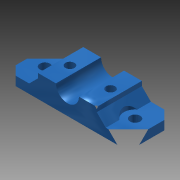
# Autodesk Inventor part: ZAxisRodClampBody
Saved by Autodesk Inventor 2015 SP1 (Build 190203100, 203)
## iProperties
Created: 2014-08-22
Part Number: ZAxisRodClampBody
Material: ABS Plastic
Document SubType Name: Modeling
Designer: t_clevj
Density: 1.06 g/cm^3
Appearance: Cyan
Mass: 6.86404 g
Surface Area: 36.706 cm^2
Volume: 6.47551 cm^3
Author: t_clevj
Autodesk Inventor part; units mm, degrees
ref_plane "YZ Plane" through (0, 0, 0) normal (1, 0, 0) x (0, 1, 0)
ref_plane "XZ Plane" through (0, 0, 0) normal (0, 1, 0) x (-1, 0, 0)
ref_plane "XY Plane" through (0, 0, 0) normal (0, 0, 1) x (1, 0, 0)
sketch "Sketch1" plane through (0, 0, 0) normal (0, 0, 1) x (1, 0, 0)
  circle A0 centre (0, 0) radius 2.25
  circle A1 centre (40, 0) radius 2.25
  line L0 (-7, 10) -> (47, 10)
  line L1 (-7, -10) -> (47, -10)
  line L2 (-7, -10) -> (-7, 10)
  line L3 (47, 10) -> (47, -10)
  dimension "d0" = 4.5
  dimension "d1" = 4.5
  dimension "d2" = 40
  dimension "d48" = 7
  dimension "d49" = 7
  dimension "d50" = 20
  dimension "d51" = 10
  constraints: 8 end point, 2 centre point, 2 perpendicular, 2 vertical, 1 coincident, 1 horizontal alignment
  measures "d0" diameter of A0
  measures "d1" diameter of A1
  measures "d2" distance of A1.centre point (0, 0)
  measures "d48" distance from line of A1.centre L3
  measures "d49" distance from line of L2 point (0, 0)
  measures "d50" distance between parallel lines of L1 L0
  measures "d51" distance from line of L0 A1.centre
extrude "Extrusion1" add sketch "Sketch1" along normal blind 4
ref_plane "Work Plane1" through (-7, 0, 0) normal (0, 1, 0) x (1, 0, 0)
sketch "Sketch4" plane through (-7, 0, 0) normal (0, 1, 0) x (1, 0, 0)
  line L0 (0, 0) -> (54, 0) projected
  line L1 (0, 0) -> (0, -4) projected
  line L2 (54, -4) -> (0, -4) projected
  line L3 (54, 0) -> (54, -4) projected
  line L4 (0, 0) -> (0, 0) projected
  line L5 (0, 0) -> (0, -4) projected
  line L6 (0, -4) -> (0, -4) projected
  line L7 (0, 0) -> (0, -4) projected
  line L8 (40, 0) -> (40, 0) projected
  line L9 (40, 0) -> (40, -4) projected
  line L10 (40, -4) -> (40, -4) projected
  line L11 (40, 0) -> (40, -4) projected
  circle A0 centre (27, -10) radius 5.1
  line L12 (14, -4) -> (14, -10)
  line L13 (14, -10) -> (21.9, -10)
  line L14 (32.1, -10) -> (40, -10)
  line L15 (40, -10) -> (40, -4)
  line L16 (0, -4) -> (54, -4) projected
  line L17 (14, -4) -> (40, -4)
  point P0 (7, 0)
  dimension "d23" = 10.2
  dimension "d24" = 6
  dimension "d25" = 26
  dimension "d26" = 13
  dimension "d27" = 14
  constraints: 10 end point, 4 point on line, 2 perpendicular, 2 point on circle, 1 centre point, 1 collinear, 1 horizontal alignment, 1 vertical
  measures "d23" diameter of A0
  measures "d24" distance from line of L2 A0.centre
  measures "d25" distance between parallel lines of L12 L15
  measures "d26" distance from line of A0.centre L15
  measures "d27" distance between parallel lines of L3 L15
extrude "Extrusion4" add sketch "Sketch4" along normal mid plane 20 contours L15 L14 A0 L13 L12 L2
chamfer "Chamfer1" distance 4 angle 45 2 edges at (7, 0, 4) (33, 0, 4)
sketch "Sketch5" plane through (0, 0, 4) normal (0, 0, 1) x (1, 0, 0)
  circle A0 centre (40, 0) radius 2.25 projected
  line L0 (3, 10) -> (-7, 10) projected
  line L1 (-7, -10) -> (3, -10) projected
  circle A1 centre (0, 0) radius 2.25 projected
  circle A2 centre (0, 0) radius 5
  circle A3 centre (40, 0) radius 2.25 projected
  circle A4 centre (40, 0) radius 5
  circle A5 centre (40, 0) radius 2.25 projected
  line L2 (47, -10) -> (47, 10) projected
  line L3 (47, 10) -> (37, 10) projected
  line L4 (-7, 10) -> (-7, -10) projected
  line L5 (37, -10) -> (37, 10) projected
  line L6 (37, -10) -> (47, -10) projected
  line L7 (3, 10) -> (3, -10) projected
  point P0 (39.5, -2.4495)
  point P1 (39.5, 2.4495)
  dimension "d33" = 10
  dimension "d34" = 10
  constraints: 2 centre point, 2 coincident, 2 other
  measures "d33" diameter of A2
  measures "d34" diameter of A4
extrude "Extrusion5" cut sketch "Sketch5" along normal up to surface (6 mm away) contours L7 A2 | A2 L7 | A1 | A4 L5 | L5 A4
sketch "Sketch6" plane through (7, 10, 10) normal (0, 0, 1) x (1, 0, 0)
  line L0 (26, -20) -> (26, 0) projected
  line L1 (18.1, 0) -> (26, 0) projected
  line L2 (18.1, -20) -> (18.1, 0) projected
  line L3 (26, -20) -> (18.1, -20) projected
  circle A0 centre (4.1, -10) radius 2
  circle A1 centre (22.1, -10) radius 2
  point P0 (-7, -10)
  dimension "d37" = 4
  dimension "d38" = 4
  dimension "d39" = 10
  dimension "d40" = 18
  dimension "d41" = 4
  constraints: 2 centre point, 1 horizontal alignment
  measures "d37" diameter of A0
  measures "d38" diameter of A1
  measures "d39" distance from line of L3 A1.centre
  measures "d40" distance of A0.centre A1.centre
  measures "d41" distance from line of L2 A1.centre
extrude "Extrusion6" cut sketch "Sketch6" against normal up to surface (10 mm away) contours A0 | A1
sketch "Sketch7" plane through (0, 0, 0) normal (0, 0, -1) x (-1, 0, 0)
  circle A0 centre (-11.1, 0) radius 2 projected
  circle A1 centre (-29.1, 0) radius 2 projected
  line L0 (-29.1, 4.2724) -> (-25.4, 2.1362)
  line L1 (-25.4, 2.1362) -> (-25.4, -2.1362)
  line L2 (-25.4, -2.1362) -> (-29.1, -4.2724)
  line L3 (-29.1, -4.2724) -> (-32.8, -2.1362)
  line L4 (-32.8, -2.1362) -> (-32.8, 2.1362)
  line L5 (-32.8, 2.1362) -> (-29.1, 4.2724)
  line L6 (-11.1, 4.2724) -> (-7.4, 2.1362)
  line L7 (-7.4, 2.1362) -> (-7.4, -2.1362)
  line L8 (-7.4, -2.1362) -> (-11.1, -4.2724)
  line L9 (-11.1, -4.2724) -> (-14.8, -2.1362)
  line L10 (-14.8, -2.1362) -> (-14.8, 2.1362)
  line L11 (-14.8, 2.1362) -> (-11.1, 4.2724)
  dimension "d44" = 7.4
  constraints: 24 end point, 2 coincident, 2 vertical, 1 parallel, 26 other
  measures "d44" distance between parallel lines of L4 L1
extrude "Extrusion7" cut sketch "Sketch7" against normal blind 3.5
chamfer "Chamfer2" distance 4 angle 45 4 edges at (-7, 10, 2) (-7, -10, 2) (47, 10, 2) (47, -10, 2)
body "Solid1"
